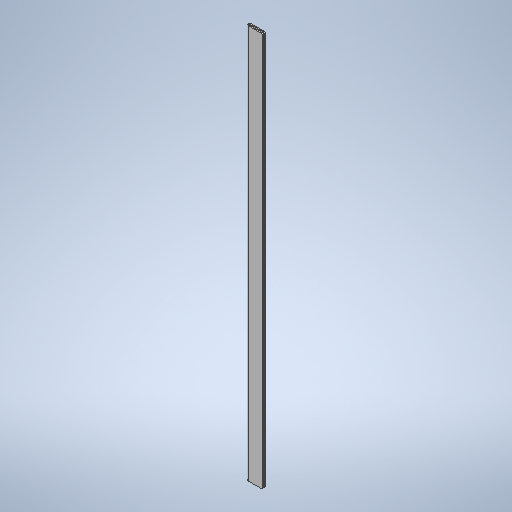
# Autodesk Inventor part: Binder
Saved by Autodesk Inventor 2025 (Build 290162000, 162)
## iProperties
Created: 2024-07-09
Part Number: Binder
Material: Generic
Document SubType Name: Modeling
Designer: usaid
Density: 1 g/cm^3
Appearance: Default
Author: usaid
Autodesk Inventor part; units mm, degrees
ref_plane "YZ Plane" through (0, 0, 0) normal (1, 0, 0) x (0, 1, 0)
ref_plane "XZ Plane" through (0, 0, 0) normal (0, 1, 0) x (-1, 0, 0)
ref_plane "XY Plane" through (0, 0, 0) normal (0, 0, 1) x (1, 0, 0)
sketch "Sketch1" plane through (0, 0, 0) normal (0, 1, 0) x (-1, 0, 0)
  arc A0 (0, -0.5) -> (0, 0.5) centre (0, 0) ccw
  arc A1 (0, -1.5) -> (0, 1.5) centre (0, 0) ccw
  line L0 (-13.5, -0.5) -> (0, -0.5)
  line L1 (-13.5, 0.5) -> (0, 0.5)
  line L2 (-13.5, -1.5) -> (0, -1.5)
  line L3 (-13.5, 1.5) -> (0, 1.5)
  line L4 (-13.5, -0.5) -> (-13.5, -1.5)
  line L5 (-13.5, 0.5) -> (-13.5, 1.5)
  constraints: 12 end point, 4 point on circle, 2 centre point
extrude "Extrusion1" add sketch "Sketch1" along normal mid plane 371.8
fillet "Fillet1" radius 1 4 edges at (13.5, 185.9, 1) (13.5, -185.9, 1) (13.5, 185.9, -1) (13.5, -185.9, -1)
body "Solid1"
